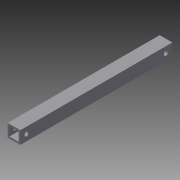
# Autodesk Inventor part: ShortBox
Saved by Autodesk Inventor 2013 (Build 170138000, 138)
## iProperties
Created: 2013-10-10
Part Number: ShortBox
Material: Gold
Document SubType Name: Modeling
Designer: cobrooks
Density: 1 g/cm^3
Author: cobrooks
Autodesk Inventor part; units mm, degrees
ref_plane "YZ Plane" through (0, 0, 0) normal (1, 0, 0) x (0, 1, 0)
ref_plane "XZ Plane" through (0, 0, 0) normal (0, 1, 0) x (-1, 0, 0)
ref_plane "XY Plane" through (0, 0, 0) normal (0, 0, 1) x (1, 0, 0)
sketch "Sketch1" plane through (0, 0, 0) normal (0, 0, 1) x (1, 0, 0)
  line L0 (-6.35, -6.35) -> (6.35, -6.35)
  line L1 (6.35, -6.35) -> (6.35, 6.35)
  line L2 (6.35, 6.35) -> (-6.35, 6.35)
  line L3 (-6.35, 6.35) -> (-6.35, -6.35)
  line L4 (-6.35, -6.35) -> (6.35, 6.35) construction
  line L5 (6.35, -6.35) -> (-6.35, 6.35) construction
  line L6 (4.572, 4.572) -> (-4.572, 4.572)
  line L7 (-4.572, 4.572) -> (-4.572, -4.572)
  line L8 (-4.572, -4.572) -> (4.572, -4.572)
  line L9 (4.572, -4.572) -> (4.572, 4.572)
  line L10 (4.572, 4.572) -> (-4.572, -4.572) construction
  line L11 (-4.572, 4.572) -> (4.572, -4.572) construction
  point P0 (0, 0)
  dimension "d0" = 12.7
  dimension "d1" = 12.7
  dimension "d2" = 10.922
  dimension "d3" = 10.922
  constraints: 24 end point, 4 midpoint, 4 parallel, 2 horizontal, 2 perpendicular
  measures "d0" distance of L2.end L1.end
  measures "d1" distance between parallel lines of L2 L0
  measures "d2" distance between parallel lines of L2 L8
  measures "d3" distance between parallel lines of L3 L9
extrude "Extrusion1" add sketch "Sketch1" along normal blind 152.4
sketch "Sketch2" plane through (6.35, -6.35, 0) normal (1, 0, 0) x (0, 0, -1)
  line L0 (0, 0) -> (0, 12.7) projected
  line L1 (-152.4, 0) -> (-152.4, 12.7) projected
  circle A0 centre (-146.05, 6.35) radius 2.1336
  circle A1 centre (-6.35, 6.35) radius 2.1336
  point P0 (0, 6.35)
  dimension "d6" = 4.2672
  dimension "d7" = 6.35
  dimension "d8" = 4.2672
  dimension "d9" = 6.35
  constraints: 2 centre point
  measures "d6" diameter of A0
  measures "d7" distance from line of L1 A0.centre
  measures "d8" diameter of A1
  measures "d9" distance from line of L0 A1.centre
extrude "Extrusion2" cut sketch "Sketch2" against normal blind 12.7
body "Solid1"
